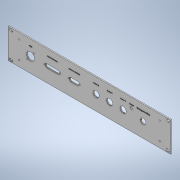
# Autodesk Inventor part: Case_Front
Saved by Autodesk Inventor 2022.2 (Build 262287010, 287A)
## iProperties
Created: 2024-11-06
Part Number: Case_Front
Material: Generisch
Document SubType Name: Modeling
Designer: ppovolni
Density: 1 g/cm^3
Appearance: Vorgabe
Author: ppovolni
Autodesk Inventor part; units mm, degrees
(part 1 of 3)
ref_plane "YZ Plane" through (0, 0, 0) normal (1, 0, 0) x (0, 1, 0)
ref_plane "XZ Plane" through (0, 0, 0) normal (0, 1, 0) x (-1, 0, 0)
ref_plane "XY Plane" through (0, 0, 0) normal (0, 0, 1) x (1, 0, 0)
sketch "Skizze3" plane through (0, 0, 0) normal (0, 0, 1) x (1, 0, 0)
  line L0 (241.3, -44.05) -> (-241.3, -44.05)
  line L1 (-241.3, -44.05) -> (-241.3, 44.05)
  line L2 (-241.3, 44.05) -> (241.3, 44.05)
  line L3 (241.3, 44.05) -> (241.3, -44.05)
  line L4 (241.3, -44.05) -> (-241.3, 44.05) construction
  line L5 (-241.3, -44.05) -> (241.3, 44.05) construction
  line L6 (-233.95, 38.1) -> (-231.05, 38.1) construction
  line L7 (-233.95, 34.35) -> (-231.05, 34.35)
  line L8 (-231.05, 41.85) -> (-233.95, 41.85)
  arc A0 (-233.95, 41.85) -> (-233.95, 34.35) centre (-233.95, 38.1) ccw
  arc A1 (-231.05, 34.35) -> (-231.05, 41.85) centre (-231.05, 38.1) ccw
  line L9 (0, 0) -> (-232.5, 0) construction
  line L10 (-232.5, 0) -> (-232.5, 38.1) construction
  line L11 (-232.5, 38.1) -> (0, 38.1) construction
  line L12 (0, 38.1) -> (0, 0) construction
  line L13 (0, 0) -> (-208.683, 0) construction
  line L14 (-208.683, 0) -> (-208.683, 26.542) construction
  line L15 (-208.683, 26.542) -> (0, 26.542) construction
  line L16 (0, 26.542) -> (0, 0) construction
  circle A2 centre (-208.683, 26.542) radius 1.7
  line L17 (0, 101) -> (0, -128) construction
  line L18 (-346, 0) -> (276, 0) construction
  line L19 (233.95, 34.35) -> (231.05, 34.35)
  line L20 (231.05, 41.85) -> (233.95, 41.85)
  arc A3 (233.95, 34.35) -> (233.95, 41.85) centre (233.95, 38.1) ccw
  arc A4 (231.05, 41.85) -> (231.05, 34.35) centre (231.05, 38.1) ccw
  circle A5 centre (208.683, 26.542) radius 1.7
  line L21 (-233.95, -38.1) -> (-231.05, -38.1) construction
  line L22 (-233.95, -34.35) -> (-231.05, -34.35)
  line L23 (-231.05, -41.85) -> (-233.95, -41.85)
  arc A6 (-233.95, -34.35) -> (-233.95, -41.85) centre (-233.95, -38.1) ccw
  arc A7 (-231.05, -41.85) -> (-231.05, -34.35) centre (-231.05, -38.1) ccw
  circle A8 centre (-208.683, -26.542) radius 1.7
  arc A9 (233.95, -41.85) -> (233.95, -34.35) centre (233.95, -38.1) ccw
  arc A10 (231.05, -34.35) -> (231.05, -41.85) centre (231.05, -38.1) ccw
  line L24 (231.05, -41.85) -> (233.95, -41.85)
  line L25 (233.95, -34.35) -> (231.05, -34.35)
  circle A11 centre (208.683, -26.542) radius 1.7
  point P0 (0, 0)
  point P1 (0, 0)
  point P2 (-227.3, 38.1)
  point P3 (-237.7, 38.1)
  point P4 (-227.3, -38.1)
  point P5 (-237.7, -38.1)
  point P6 (-232.5, -38.1)
  dimension "d0" = 482.6
  dimension "d1" = 88.1
  dimension "d6" = 7.5
  dimension "d7" = 10.4
  dimension "d8" = 38.1
  dimension "d9" = 232.5
  dimension "d10" = 3.4
  dimension "d11" = 208.683
  dimension "d12" = 26.542
  constraints: 56 end point, 25 symmetric about line, 18 point on circle, 12 centre point, 7 parallel, 5 horizontal, 5 midpoint, 4 tangent, 3 perpendicular, 2 coincident, 2 point on line, 1 vertical, 9 other
  measures "d0" distance of L1.end L2.end
  measures "d1" distance of L0.end L1.end
  measures "d6" distance between parallel lines of L7 L8
  measures "d7" distance of point (-227.3, 38.1) point (-237.7, 38.1)
  measures "d8" distance of L9.end L10.end
  measures "d9" distance of L10.end L11.end
  measures "d10" diameter of A2
  measures "d11" distance of L14.end L15.end
  measures "d12" distance of L13.end L14.end
extrude "Extrusion1" add sketch "Skizze3" along normal blind 3
sketch "Skizze4" plane through (0, 0, 3) normal (0, 0, 1) x (1, 0, 0)
  line L0 (241.3, 44.05) -> (-241.3, 44.05) construction
  line L1 (-241.3, 44.05) -> (-241.3, -44.05) construction
  line L2 (-241.3, -44.05) -> (241.3, -44.05) construction
  line L3 (241.3, -44.05) -> (241.3, 44.05) construction
  circle A0 centre (-208.683, 26.542) radius 1.7 construction
  circle A1 centre (208.683, 26.542) radius 1.7 construction
  circle A2 centre (-208.683, -26.542) radius 1.7 construction
  circle A3 centre (208.683, -26.542) radius 1.7 construction
  line L4 (231.05, -34.35) -> (233.95, -34.35) construction
  arc A4 (233.95, -41.85) -> (233.95, -34.35) centre (233.95, -38.1) ccw construction
  line L5 (233.95, -41.85) -> (231.05, -41.85) construction
  arc A5 (231.05, -34.35) -> (231.05, -41.85) centre (231.05, -38.1) ccw construction
  line L6 (-233.95, -34.35) -> (-231.05, -34.35) construction
  arc A6 (-231.05, -41.85) -> (-231.05, -34.35) centre (-231.05, -38.1) ccw construction
  line L7 (-231.05, -41.85) -> (-233.95, -41.85) construction
  arc A7 (-233.95, -34.35) -> (-233.95, -41.85) centre (-233.95, -38.1) ccw construction
  line L8 (231.05, 41.85) -> (233.95, 41.85) construction
  arc A8 (233.95, 34.35) -> (233.95, 41.85) centre (233.95, 38.1) ccw construction
  line L9 (233.95, 34.35) -> (231.05, 34.35) construction
  arc A9 (231.05, 41.85) -> (231.05, 34.35) centre (231.05, 38.1) ccw construction
  arc A10 (-233.95, 41.85) -> (-233.95, 34.35) centre (-233.95, 38.1) ccw construction
  line L10 (-233.95, 41.85) -> (-231.05, 41.85) construction
  arc A11 (-231.05, 34.35) -> (-231.05, 41.85) centre (-231.05, 38.1) ccw construction
  line L11 (-231.05, 34.35) -> (-233.95, 34.35) construction
  circle A12 centre (-175, 0) radius 11.8
  line L12 (-184.5, -12) -> (-165.5, -12) construction
  line L13 (-165.5, -12) -> (-165.5, 12) construction
  line L14 (-165.5, 12) -> (-184.5, 12) construction
  line L15 (-184.5, 12) -> (-184.5, -12) construction
  line L16 (-184.5, -12) -> (-165.5, 12) construction
  line L17 (-165.5, -12) -> (-184.5, 12) construction
  circle A13 centre (-165.5, 12) radius 1.55
  circle A14 centre (-184.5, -12) radius 1.55
  line L18 (-128.2985, 5) -> (-91.7015, 5)
  line L19 (-89.2395, 2.0659) -> (-90.1211, -2.9341)
  line L20 (-92.5832, -5) -> (-127.4168, -5)
  line L21 (-129.8789, -2.9341) -> (-130.7605, 2.0659)
  line L22 (-131.2779, 5) -> (-88.7221, 5) construction
  line L23 (-88.7221, 5) -> (-88.7221, -5) construction
  line L24 (-88.7221, -5) -> (-131.2779, -5) construction
  line L25 (-131.2779, -5) -> (-131.2779, 5) construction
  line L26 (-110, -5) -> (-110, 5) construction
  line L27 (-131.2779, 0) -> (-88.7221, 0) construction
  circle A15 centre (-133.52, 0) radius 1.55
  circle A16 centre (-86.48, 0) radius 1.55
  arc A17 (-128.2985, 5) -> (-130.7605, 2.0659) centre (-128.2985, 2.5) ccw
  arc A18 (-129.8789, -2.9341) -> (-127.4168, -5) centre (-127.4168, -2.5) ccw
  arc A19 (-89.2395, 2.0659) -> (-91.7015, 5) centre (-91.7015, 2.5) ccw
  arc A20 (-92.5832, -5) -> (-90.1211, -2.9341) centre (-92.5832, -2.5) ccw
  line L28 (-56.638, 5.6) -> (-33.362, 5.6)
  line L29 (-30.9, 2.6659) -> (-31.9932, -3.5341)
  line L30 (-34.4552, -5.6) -> (-55.5448, -5.6)
  line L31 (-58.0068, -3.5341) -> (-59.1, 2.6659)
  line L32 (-59.6174, 5.6) -> (-30.3826, 5.6) construction
  line L33 (-30.3826, 5.6) -> (-30.3826, -5.6) construction
  line L34 (-30.3826, -5.6) -> (-59.6174, -5.6) construction
  line L35 (-59.6174, -5.6) -> (-59.6174, 5.6) construction
  line L36 (-45, -5.6) -> (-45, 5.6) construction
  line L37 (-59.6174, 0) -> (-30.3826, 0) construction
  circle A21 centre (-61.66, 0) radius 1.55
  circle A22 centre (-28.34, 0) radius 1.55
  arc A23 (-56.638, 5.6) -> (-59.1, 2.6659) centre (-56.638, 3.1) ccw
  arc A24 (-58.0068, -3.5341) -> (-55.5448, -5.6) centre (-55.5448, -3.1) ccw
  arc A25 (-30.9, 2.6659) -> (-33.362, 5.6) centre (-33.362, 3.1) ccw
  arc A26 (-34.4552, -5.6) -> (-31.9932, -3.5341) centre (-34.4552, -3.1) ccw
  arc A27 (21.536, -8.868) -> (18.464, -8.868) centre (20, 0) ccw
  line L38 (20, 9.0139) -> (20, -9.0139) construction
  line L39 (11, 0) -> (29, 0) construction
  line L40 (20, -8.2) -> (20, -10.3) construction
  arc A28 (21.536, -8.868) -> (18.464, -8.868) centre (20, -10.3) ccw
  arc A29 (61.536, -8.868) -> (58.464, -8.868) centre (60, 0) ccw
  line L41 (60, 31.8347) -> (60, -31.8347) construction
  line L42 (51, 0) -> (69, 0) construction
  line L43 (60, -8.2) -> (60, -10.3) construction
  arc A30 (61.536, -8.868) -> (58.464, -8.868) centre (60, -10.3) ccw
  arc A31 (101.536, -8.868) -> (98.464, -8.868) centre (100, 0) ccw
  line L44 (100, 22.1437) -> (100, -22.1437) construction
  line L45 (91, 0) -> (109, 0) construction
  line L46 (100, -8.2) -> (100, -10.3) construction
  arc A32 (101.536, -8.868) -> (98.464, -8.868) centre (100, -10.3) ccw
  circle A33 centre (125, 17) radius 4
  line L47 (-241.3, 19.05) -> (241.3, 19.05) construction
  line L48 (-180, 19.05) -> (-170, 19.05) construction
  line L49 (-170, 19.05) -> (-170, 24.05) construction
  line L50 (-170, 24.05) -> (-180, 24.05) construction
  line L51 (-180, 24.05) -> (-180, 19.05) construction
  line L52 (-115, 19.05) -> (-105, 19.05) construction
  line L53 (-105, 19.05) -> (-105, 24.05) construction
  line L54 (-105, 24.05) -> (-115, 24.05) construction
  line L55 (-115, 24.05) -> (-115, 19.05) construction
  line L56 (-50, 19.05) -> (-40, 19.05) construction
  line L57 (-40, 19.05) -> (-40, 24.05) construction
  line L58 (-40, 24.05) -> (-50, 24.05) construction
  line L59 (-50, 24.05) -> (-50, 19.05) construction
  line L60 (15, 19.05) -> (25, 19.05) construction
  line L61 (25, 19.05) -> (25, 24.05) construction
  line L62 (25, 24.05) -> (15, 24.05) construction
  line L63 (15, 24.05) -> (15, 19.05) construction
  line L64 (55, 19.05) -> (65, 19.05) construction
  line L65 (65, 19.05) -> (65, 24.05) construction
  line L66 (65, 24.05) -> (55, 24.05) construction
  line L67 (55, 24.05) -> (55, 19.05) construction
  line L68 (95, 19.05) -> (105, 19.05) construction
  line L69 (105, 19.05) -> (105, 24.05) construction
  line L70 (105, 24.05) -> (95, 24.05) construction
  line L71 (95, 24.05) -> (95, 19.05) construction
  line L72 (120, 19.05) -> (130, 19.05) construction
  line L73 (130, 19.05) -> (130, 24.05) construction
  line L74 (130, 24.05) -> (120, 24.05) construction
  line L75 (120, 24.05) -> (120, 19.05) construction
  arc A34 (151.5453, -0.85) -> (151.5453, 0.85) centre (159.5, 0) ccw
  line L76 (152.5, 0) -> (167.5, 0) construction
  line L77 (167.4657, 0.7397) -> (167.4657, -0.7397) construction
  line L78 (151.5453, 0.85) -> (152.5, 0.85)
  line L79 (152.5, 0.85) -> (152.5, -0.85)
  line L80 (152.5, -0.85) -> (151.5453, -0.85)
  line L81 (155, 19.05) -> (165, 19.05) construction
  line L82 (165, 19.05) -> (165, 24.05) construction
  line L83 (165, 24.05) -> (155, 24.05) construction
  line L84 (155, 24.05) -> (155, 19.05) construction
  spline S0 degree 2 poles (-177.7216, 23.9868) (-178.327, 23.9868) (-178.9785, 24.5703) (-178.9785, 25.1343) knots 0 0 0 1 2 2 2
  line L85 (-178.9785, 25.1343) -> (-178.9785, 27.05)
  line L86 (-178.9785, 27.05) -> (-178.2249, 27.05)
  line L87 (-178.2249, 27.05) -> (-178.2249, 25.178)
  spline S1 degree 2 poles (-178.2249, 25.178) (-178.2249, 24.8644) (-177.9891, 24.5581) (-177.7216, 24.5581) knots 0 0 0 1 2 2 2
  spline S2 degree 2 poles (-177.7216, 24.5581) (-177.4615, 24.5581) (-177.2184, 24.8523) (-177.2184, 25.178) knots 0 0 0 1 2 2 2
  line L88 (-177.2184, 25.178) -> (-177.2184, 27.05)
  line L89 (-177.2184, 27.05) -> (-176.4647, 27.05)
  line L90 (-176.4647, 27.05) -> (-176.4647, 25.1367)
  spline S3 degree 2 poles (-176.4647, 25.1367) (-176.4647, 24.5824) (-177.0993, 23.9868) (-177.7216, 23.9868) knots 0 0 0 1 2 2 2
  spline S4 degree 2 poles (-174.9599, 23.9965) (-175.3051, 23.9965) (-175.8254, 24.1302) (-176.049, 24.2275) knots 0 0 0 1 2 2 2
  line L91 (-176.049, 24.2275) -> (-176.049, 24.9422)
  line L92 (-176.049, 24.9422) -> (-175.981, 24.9422)
  spline S5 degree 2 poles (-175.981, 24.9422) (-175.7549, 24.7502) (-175.2127, 24.5435) (-174.9575, 24.5435) knots 0 0 0 1 2 2 2
  spline S6 degree 2 poles (-174.9575, 24.5435) (-174.8918, 24.5435) (-174.6803, 24.5727) (-174.6171, 24.6019) knots 0 0 0 1 2 2 2
  spline S7 degree 2 poles (-174.6171, 24.6019) (-174.5393, 24.6359) (-174.4299, 24.7599) (-174.4299, 24.8596) knots 0 0 0 1 2 2 2
  spline S8 degree 2 poles (-174.4299, 24.8596) (-174.4299, 24.9738) (-174.6074, 25.1148) (-174.7289, 25.1464) knots 0 0 0 1 2 2 2
  spline S9 degree 2 poles (-174.7289, 25.1464) (-174.8821, 25.1878) (-175.2297, 25.2583) (-175.3829, 25.3118) knots 0 0 0 1 2 2 2
  spline S10 degree 2 poles (-175.3829, 25.3118) (-175.7306, 25.4333) (-176.032, 25.849) (-176.032, 26.1602) knots 0 0 0 1 2 2 2
  spline S11 degree 2 poles (-176.032, 26.1602) (-176.032, 26.5808) (-175.3197, 27.1035) (-174.7848, 27.1035) knots 0 0 0 1 2 2 2
  spline S12 degree 2 poles (-174.7848, 27.1035) (-174.5174, 27.1035) (-173.9874, 26.9941) (-173.7784, 26.9017) knots 0 0 0 1 2 2 2
  line L93 (-173.7784, 26.9017) -> (-173.7784, 26.2161)
  line L94 (-173.7784, 26.2161) -> (-173.844, 26.2161)
  spline S13 degree 2 poles (-173.844, 26.2161) (-174.0118, 26.3596) (-174.4931, 26.5565) (-174.7459, 26.5565) knots 0 0 0 1 2 2 2
  spline S14 degree 2 poles (-174.7459, 26.5565) (-174.8456, 26.5565) (-175.0012, 26.5273) (-175.0887, 26.4884) knots 0 0 0 1 2 2 2
  spline S15 degree 2 poles (-175.0887, 26.4884) (-175.1592, 26.4568) (-175.2613, 26.3304) (-175.2613, 26.2526) knots 0 0 0 1 2 2 2
  spline S16 degree 2 poles (-175.2613, 26.2526) (-175.2613, 26.1359) (-175.0985, 26.0022) (-174.8651, 25.9487) knots 0 0 0 1 2 2 2
  spline S17 degree 2 poles (-174.8651, 25.9487) (-174.7143, 25.9147) (-174.4348, 25.849) (-174.2743, 25.7931) knots 0 0 0 1 2 2 2
  spline S18 degree 2 poles (-174.2743, 25.7931) (-173.9631, 25.6788) (-173.6592, 25.2996) (-173.6592, 24.9884) knots 0 0 0 1 2 2 2
  spline S19 degree 2 poles (-173.6592, 24.9884) (-173.6592, 24.5411) (-174.3618, 23.9965) (-174.9599, 23.9965) knots 0 0 0 1 2 2 2
  spline S20 degree 2 poles (-170.8756, 24.969) (-170.8756, 24.7453) (-171.0458, 24.4074) (-171.1868, 24.2955) knots 0 0 0 1 2 2 2
  spline S21 degree 2 poles (-171.1868, 24.2955) (-171.357, 24.1618) (-171.7605, 24.05) (-172.0741, 24.05) knots 0 0 0 1 2 2 2
  line L95 (-172.0741, 24.05) -> (-173.2727, 24.05)
  line L96 (-173.2727, 24.05) -> (-173.2727, 27.05)
  line L97 (-173.2727, 27.05) -> (-172.2152, 27.05)
  spline S22 degree 2 poles (-172.2152, 27.05) (-171.8845, 27.05) (-171.5442, 26.9989) (-171.3959, 26.9187) knots 0 0 0 1 2 2 2
  spline S23 degree 2 poles (-171.3959, 26.9187) (-171.233, 26.8336) (-171.075, 26.5419) (-171.075, 26.3523) knots 0 0 0 1 2 2 2
  spline S24 degree 2 poles (-171.075, 26.3523) (-171.075, 26.1335) (-171.2938, 25.7907) (-171.4882, 25.7105) knots 0 0 0 1 2 2 2
  line L98 (-171.4882, 25.7105) -> (-171.4882, 25.6959)
  spline S25 degree 2 poles (-171.4882, 25.6959) (-171.2087, 25.6375) (-170.8756, 25.2753) (-170.8756, 24.969) knots 0 0 0 1 2 2 2
  spline S26 degree 2 poles (-171.6536, 24.9811) (-171.6536, 25.1221) (-171.7654, 25.2801) (-171.8772, 25.3215) knots 0 0 0 1 2 2 2
  spline S27 degree 2 poles (-171.8772, 25.3215) (-171.9453, 25.3482) (-172.186, 25.3531) (-172.3853, 25.3531) knots 0 0 0 1 2 2 2
  line L99 (-172.3853, 25.3531) -> (-172.5239, 25.3531)
  line L100 (-172.5239, 25.3531) -> (-172.5239, 24.597)
  line L101 (-172.5239, 24.597) -> (-172.4826, 24.597)
  spline S28 degree 2 poles (-172.4826, 24.597) (-172.1908, 24.597) (-171.9672, 24.6043) (-171.8505, 24.6553) knots 0 0 0 1 2 2 2
  spline S29 degree 2 poles (-171.8505, 24.6553) (-171.7484, 24.7015) (-171.6536, 24.8717) (-171.6536, 24.9811) knots 0 0 0 1 2 2 2
  spline S30 degree 2 poles (-171.8408, 26.204) (-171.8408, 26.2769) (-171.9161, 26.4301) (-171.9939, 26.4641) knots 0 0 0 1 2 2 2
  spline S31 degree 2 poles (-171.9939, 26.4641) (-172.0669, 26.4981) (-172.2711, 26.503) (-172.4729, 26.503) knots 0 0 0 1 2 2 2
  line L102 (-172.4729, 26.503) -> (-172.5239, 26.503)
  line L103 (-172.5239, 26.503) -> (-172.5239, 25.866)
  line L104 (-172.5239, 25.866) -> (-172.4291, 25.866)
  spline S32 degree 2 poles (-172.4291, 25.866) (-172.237, 25.866) (-172.0814, 25.8733) (-171.9988, 25.9122) knots 0 0 0 1 2 2 2
  spline S33 degree 2 poles (-171.9988, 25.9122) (-171.9088, 25.956) (-171.8408, 26.1043) (-171.8408, 26.204) knots 0 0 0 1 2 2 2
  line L105 (-122.857, 24.05) -> (-124.8578, 24.05)
  line L106 (-124.8578, 24.05) -> (-124.8578, 27.05)
  line L107 (-124.8578, 27.05) -> (-124.1041, 27.05)
  line L108 (-124.1041, 27.05) -> (-124.1041, 24.6213)
  line L109 (-124.1041, 24.6213) -> (-122.857, 24.6213)
  line L110 (-122.857, 24.6213) -> (-122.857, 24.05)
  line L111 (-121.8335, 24.05) -> (-122.5385, 24.05)
  line L112 (-122.5385, 24.05) -> (-122.5385, 26.3134)
  line L113 (-122.5385, 26.3134) -> (-121.8335, 26.3134)
  line L114 (-121.8335, 26.3134) -> (-121.8335, 24.05)
  line L115 (-121.8116, 26.6367) -> (-122.5579, 26.6367)
  line L116 (-122.5579, 26.6367) -> (-122.5579, 27.1861)
  line L117 (-122.5579, 27.1861) -> (-121.8116, 27.1861)
  line L118 (-121.8116, 27.1861) -> (-121.8116, 26.6367)
  line L119 (-118.5928, 24.05) -> (-118.5928, 25.1805)
  spline S34 degree 2 poles (-118.5928, 25.1805) (-118.5928, 25.3482) (-118.6049, 25.5767) (-118.6341, 25.6497) knots 0 0 0 1 2 2 2
  spline S35 degree 2 poles (-118.6341, 25.6497) (-118.6657, 25.7226) (-118.7921, 25.7882) (-118.9064, 25.7882) knots 0 0 0 1 2 2 2
  spline S36 degree 2 poles (-118.9064, 25.7882) (-118.9866, 25.7882) (-119.1422, 25.7177) (-119.2346, 25.6521) knots 0 0 0 1 2 2 2
  line L120 (-119.2346, 25.6521) -> (-119.2346, 24.05)
  line L121 (-119.2346, 24.05) -> (-119.9445, 24.05)
  line L122 (-119.9445, 24.05) -> (-119.9445, 25.1805)
  spline S37 degree 2 poles (-119.9445, 25.1805) (-119.9445, 25.3458) (-119.9591, 25.5767) (-119.9883, 25.6497) knots 0 0 0 1 2 2 2
  spline S38 degree 2 poles (-119.9883, 25.6497) (-120.0199, 25.7226) (-120.1463, 25.7882) (-120.2605, 25.7882) knots 0 0 0 1 2 2 2
  spline S39 degree 2 poles (-120.2605, 25.7882) (-120.3456, 25.7882) (-120.5134, 25.708) (-120.5912, 25.6521) knots 0 0 0 1 2 2 2
  line L123 (-120.5912, 25.6521) -> (-120.5912, 24.05)
  line L124 (-120.5912, 24.05) -> (-121.2962, 24.05)
  line L125 (-121.2962, 24.05) -> (-121.2962, 26.3134)
  line L126 (-121.2962, 26.3134) -> (-120.5912, 26.3134)
  line L127 (-120.5912, 26.3134) -> (-120.5912, 26.063)
  spline S40 degree 2 poles (-120.5912, 26.063) (-120.4186, 26.2088) (-120.1098, 26.3741) (-119.9177, 26.3741) knots 0 0 0 1 2 2 2
  spline S41 degree 2 poles (-119.9177, 26.3741) (-119.7111, 26.3741) (-119.3951, 26.1772) (-119.3124, 25.9803) knots 0 0 0 1 2 2 2
  spline S42 degree 2 poles (-119.3124, 25.9803) (-119.1106, 26.1699) (-118.7508, 26.3741) (-118.566, 26.3741) knots 0 0 0 1 2 2 2
  spline S43 degree 2 poles (-118.566, 26.3741) (-118.408, 26.3741) (-118.1576, 26.2745) (-118.0725, 26.1724) knots 0 0 0 1 2 2 2
  spline S44 degree 2 poles (-118.0725, 26.1724) (-117.9777, 26.063) (-117.8829, 25.7639) (-117.8829, 25.5233) knots 0 0 0 1 2 2 2
  line L128 (-117.8829, 25.5233) -> (-117.8829, 24.05)
  line L129 (-117.8829, 24.05) -> (-118.5928, 24.05)
  line L130 (-116.6552, 24.05) -> (-117.3602, 24.05)
  line L131 (-117.3602, 24.05) -> (-117.3602, 26.3134)
  line L132 (-117.3602, 26.3134) -> (-116.6552, 26.3134)
  line L133 (-116.6552, 26.3134) -> (-116.6552, 24.05)
  line L134 (-116.6333, 26.6367) -> (-117.3797, 26.6367)
  line L135 (-117.3797, 26.6367) -> (-117.3797, 27.1861)
  line L136 (-117.3797, 27.1861) -> (-116.6333, 27.1861)
  line L137 (-116.6333, 27.1861) -> (-116.6333, 26.6367)
  spline S45 degree 2 poles (-115.25, 24.0062) (-115.6803, 24.0062) (-116.0741, 24.3612) (-116.0741, 24.7647) knots 0 0 0 1 2 2 2
  line L138 (-116.0741, 24.7647) -> (-116.0741, 25.8223)
  line L139 (-116.0741, 25.8223) -> (-116.344, 25.8223)
  line L140 (-116.344, 25.8223) -> (-116.344, 26.3134)
  line L141 (-116.344, 26.3134) -> (-116.0741, 26.3134)
  line L142 (-116.0741, 26.3134) -> (-116.0741, 26.96)
  line L143 (-116.0741, 26.96) -> (-115.3691, 26.96)
  line L144 (-115.3691, 26.96) -> (-115.3691, 26.3134)
  line L145 (-115.3691, 26.3134) -> (-114.6884, 26.3134)
  line L146 (-114.6884, 26.3134) -> (-114.6884, 25.8223)
  line L147 (-114.6884, 25.8223) -> (-115.3691, 25.8223)
  line L148 (-115.3691, 25.8223) -> (-115.3691, 25.0176)
  spline S46 degree 2 poles (-115.3691, 25.0176) (-115.3691, 24.8985) (-115.3643, 24.721) (-115.3351, 24.6505) knots 0 0 0 1 2 2 2
  spline S47 degree 2 poles (-115.3351, 24.6505) (-115.3059, 24.58) (-115.1625, 24.4973) (-115.0263, 24.4973) knots 0 0 0 1 2 2 2
  spline S48 degree 2 poles (-115.0263, 24.4973) (-114.968, 24.4973) (-114.7857, 24.5459) (-114.7492, 24.5654) knots 0 0 0 1 2 2 2
  line L149 (-114.7492, 24.5654) -> (-114.6884, 24.5654)
  line L150 (-114.6884, 24.5654) -> (-114.6884, 24.0694)
  spline S49 degree 2 poles (-114.6884, 24.0694) (-114.8027, 24.0403) (-115.0604, 24.0062) (-115.25, 24.0062) knots 0 0 0 1 2 2 2
  spline S50 degree 2 poles (-112.2257, 23.9965) (-112.5709, 23.9965) (-113.0912, 24.1302) (-113.3148, 24.2275) knots 0 0 0 1 2 2 2
  line L151 (-113.3148, 24.2275) -> (-113.3148, 24.9422)
  line L152 (-113.3148, 24.9422) -> (-113.2468, 24.9422)
  spline S51 degree 2 poles (-113.2468, 24.9422) (-113.0207, 24.7502) (-112.4785, 24.5435) (-112.2233, 24.5435) knots 0 0 0 1 2 2 2
  spline S52 degree 2 poles (-112.2233, 24.5435) (-112.1576, 24.5435) (-111.9461, 24.5727) (-111.8829, 24.6019) knots 0 0 0 1 2 2 2
  spline S53 degree 2 poles (-111.8829, 24.6019) (-111.8051, 24.6359) (-111.6957, 24.7599) (-111.6957, 24.8596) knots 0 0 0 1 2 2 2
  spline S54 degree 2 poles (-111.6957, 24.8596) (-111.6957, 24.9738) (-111.8732, 25.1148) (-111.9947, 25.1464) knots 0 0 0 1 2 2 2
  spline S55 degree 2 poles (-111.9947, 25.1464) (-112.1479, 25.1878) (-112.4955, 25.2583) (-112.6487, 25.3118) knots 0 0 0 1 2 2 2
  spline S56 degree 2 poles (-112.6487, 25.3118) (-112.9964, 25.4333) (-113.2978, 25.849) (-113.2978, 26.1602) knots 0 0 0 1 2 2 2
  spline S57 degree 2 poles (-113.2978, 26.1602) (-113.2978, 26.5808) (-112.5855, 27.1035) (-112.0506, 27.1035) knots 0 0 0 1 2 2 2
  spline S58 degree 2 poles (-112.0506, 27.1035) (-111.7832, 27.1035) (-111.2532, 26.9941) (-111.0442, 26.9017) knots 0 0 0 1 2 2 2
  line L153 (-111.0442, 26.9017) -> (-111.0442, 26.2161)
  line L154 (-111.0442, 26.2161) -> (-111.1098, 26.2161)
  spline S59 degree 2 poles (-111.1098, 26.2161) (-111.2776, 26.3596) (-111.7589, 26.5565) (-112.0118, 26.5565) knots 0 0 0 1 2 2 2
  spline S60 degree 2 poles (-112.0118, 26.5565) (-112.1114, 26.5565) (-112.267, 26.5273) (-112.3545, 26.4884) knots 0 0 0 1 2 2 2
  spline S61 degree 2 poles (-112.3545, 26.4884) (-112.425, 26.4568) (-112.5271, 26.3304) (-112.5271, 26.2526) knots 0 0 0 1 2 2 2
  spline S62 degree 2 poles (-112.5271, 26.2526) (-112.5271, 26.1359) (-112.3643, 26.0022) (-112.1309, 25.9487) knots 0 0 0 1 2 2 2
  spline S63 degree 2 poles (-112.1309, 25.9487) (-111.9801, 25.9147) (-111.7006, 25.849) (-111.5401, 25.7931) knots 0 0 0 1 2 2 2
  spline S64 degree 2 poles (-111.5401, 25.7931) (-111.2289, 25.6788) (-110.925, 25.2996) (-110.925, 24.9884) knots 0 0 0 1 2 2 2
  spline S65 degree 2 poles (-110.925, 24.9884) (-110.925, 24.5411) (-111.6276, 23.9965) (-112.2257, 23.9965) knots 0 0 0 1 2 2 2
  line L155 (-107.2079, 26.3134) -> (-107.8691, 24.05)
  line L156 (-107.8691, 24.05) -> (-108.6179, 24.05)
  line L157 (-108.6179, 24.05) -> (-109.0166, 25.5135)
  line L158 (-109.0166, 25.5135) -> (-109.4153, 24.05)
  line L159 (-109.4153, 24.05) -> (-110.1641, 24.05)
  line L160 (-110.1641, 24.05) -> (-110.8205, 26.3134)
  line L161 (-110.8205, 26.3134) -> (-110.079, 26.3134)
  line L162 (-110.079, 26.3134) -> (-109.7314, 24.8158)
  line L163 (-109.7314, 24.8158) -> (-109.3035, 26.3134)
  line L164 (-109.3035, 26.3134) -> (-108.6787, 26.3134)
  line L165 (-108.6787, 26.3134) -> (-108.2751, 24.8158)
  line L166 (-108.2751, 24.8158) -> (-107.9323, 26.3134)
  line L167 (-107.9323, 26.3134) -> (-107.2079, 26.3134)
  line L168 (-106.2038, 24.05) -> (-106.9088, 24.05)
  line L169 (-106.9088, 24.05) -> (-106.9088, 26.3134)
  line L170 (-106.9088, 26.3134) -> (-106.2038, 26.3134)
  line L171 (-106.2038, 26.3134) -> (-106.2038, 24.05)
  line L172 (-106.1819, 26.6367) -> (-106.9283, 26.6367)
  line L173 (-106.9283, 26.6367) -> (-106.9283, 27.1861)
  line L174 (-106.9283, 27.1861) -> (-106.1819, 27.1861)
  line L175 (-106.1819, 27.1861) -> (-106.1819, 26.6367)
  spline S66 degree 2 poles (-104.7986, 24.0062) (-105.2289, 24.0062) (-105.6228, 24.3612) (-105.6228, 24.7647) knots 0 0 0 1 2 2 2
  line L176 (-105.6228, 24.7647) -> (-105.6228, 25.8223)
  line L177 (-105.6228, 25.8223) -> (-105.8926, 25.8223)
  line L178 (-105.8926, 25.8223) -> (-105.8926, 26.3134)
  line L179 (-105.8926, 26.3134) -> (-105.6228, 26.3134)
  line L180 (-105.6228, 26.3134) -> (-105.6228, 26.96)
  line L181 (-105.6228, 26.96) -> (-104.9177, 26.96)
  line L182 (-104.9177, 26.96) -> (-104.9177, 26.3134)
  line L183 (-104.9177, 26.3134) -> (-104.237, 26.3134)
  line L184 (-104.237, 26.3134) -> (-104.237, 25.8223)
  line L185 (-104.237, 25.8223) -> (-104.9177, 25.8223)
  line L186 (-104.9177, 25.8223) -> (-104.9177, 25.0176)
  spline S67 degree 2 poles (-104.9177, 25.0176) (-104.9177, 24.8985) (-104.9129, 24.721) (-104.8837, 24.6505) knots 0 0 0 1 2 2 2
  spline S68 degree 2 poles (-104.8837, 24.6505) (-104.8545, 24.58) (-104.7111, 24.4973) (-104.575, 24.4973) knots 0 0 0 1 2 2 2
  spline S69 degree 2 poles (-104.575, 24.4973) (-104.5166, 24.4973) (-104.3343, 24.5459) (-104.2978, 24.5654) knots 0 0 0 1 2 2 2
  line L187 (-104.2978, 24.5654) -> (-104.237, 24.5654)
  line L188 (-104.237, 24.5654) -> (-104.237, 24.0694)
  spline S70 degree 2 poles (-104.237, 24.0694) (-104.3513, 24.0403) (-104.609, 24.0062) (-104.7986, 24.0062) knots 0 0 0 1 2 2 2
  spline S71 degree 2 poles (-102.8416, 23.9892) (-103.1211, 23.9892) (-103.5855, 24.1302) (-103.7581, 24.2761) knots 0 0 0 1 2 2 2
  spline S72 degree 2 poles (-103.7581, 24.2761) (-103.9259, 24.4244) (-104.1155, 24.8693) (-104.1155, 25.1707) knots 0 0 0 1 2 2 2
  spline S73 degree 2 poles (-104.1155, 25.1707) (-104.1155, 25.4965) (-103.9113, 25.9511) (-103.7338, 26.097) knots 0 0 0 1 2 2 2
  spline S74 degree 2 poles (-103.7338, 26.097) (-103.566, 26.238) (-103.109, 26.3741) (-102.861, 26.3741) knots 0 0 0 1 2 2 2
  spline S75 degree 2 poles (-102.861, 26.3741) (-102.6738, 26.3741) (-102.2994, 26.2866) (-102.1098, 26.1918) knots 0 0 0 1 2 2 2
  line L189 (-102.1098, 26.1918) -> (-102.1098, 25.5889)
  line L190 (-102.1098, 25.5889) -> (-102.1998, 25.5889)
  spline S76 degree 2 poles (-102.1998, 25.5889) (-102.2435, 25.6302) (-102.3651, 25.7275) (-102.438, 25.7664) knots 0 0 0 1 2 2 2
  spline S77 degree 2 poles (-102.438, 25.7664) (-102.5158, 25.8101) (-102.7079, 25.8685) (-102.827, 25.8685) knots 0 0 0 1 2 2 2
  spline S78 degree 2 poles (-102.827, 25.8685) (-103.0968, 25.8685) (-103.3934, 25.4917) (-103.3934, 25.1707) knots 0 0 0 1 2 2 2
  spline S79 degree 2 poles (-103.3934, 25.1707) (-103.3934, 24.8304) (-103.0774, 24.4949) (-102.8148, 24.4949) knots 0 0 0 1 2 2 2
  spline S80 degree 2 poles (-102.8148, 24.4949) (-102.6811, 24.4949) (-102.4818, 24.5557) (-102.4088, 24.5994) knots 0 0 0 1 2 2 2
  spline S81 degree 2 poles (-102.4088, 24.5994) (-102.3383, 24.6408) (-102.2362, 24.7331) (-102.1998, 24.7696) knots 0 0 0 1 2 2 2
  line L191 (-102.1998, 24.7696) -> (-102.1098, 24.7696)
  line L192 (-102.1098, 24.7696) -> (-102.1098, 24.1643)
  spline S82 degree 2 poles (-102.1098, 24.1643) (-102.1706, 24.1375) (-102.3286, 24.0694) (-102.4113, 24.0476) knots 0 0 0 1 2 2 2
  spline S83 degree 2 poles (-102.4113, 24.0476) (-102.5134, 24.0184) (-102.6933, 23.9892) (-102.8416, 23.9892) knots 0 0 0 1 2 2 2
  line L193 (-99.6568, 24.05) -> (-100.3667, 24.05)
  line L194 (-100.3667, 24.05) -> (-100.3667, 25.1707)
  spline S84 degree 2 poles (-100.3667, 25.1707) (-100.3667, 25.3093) (-100.3886, 25.5816) (-100.4177, 25.6448) knots 0 0 0 1 2 2 2
  spline S85 degree 2 poles (-100.4177, 25.6448) (-100.4542, 25.7226) (-100.5904, 25.7882) (-100.707, 25.7882) knots 0 0 0 1 2 2 2
  spline S86 degree 2 poles (-100.707, 25.7882) (-100.7921, 25.7882) (-100.9696, 25.7226) (-101.0693, 25.6521) knots 0 0 0 1 2 2 2
  line L195 (-101.0693, 25.6521) -> (-101.0693, 24.05)
  line L196 (-101.0693, 24.05) -> (-101.7743, 24.05)
  line L197 (-101.7743, 24.05) -> (-101.7743, 27.1837)
  line L198 (-101.7743, 27.1837) -> (-101.0693, 27.1837)
  line L199 (-101.0693, 27.1837) -> (-101.0693, 26.063)
  spline S87 degree 2 poles (-101.0693, 26.063) (-100.8967, 26.2088) (-100.5685, 26.3741) (-100.3691, 26.3741) knots 0 0 0 1 2 2 2
  spline S88 degree 2 poles (-100.3691, 26.3741) (-100.0239, 26.3741) (-99.6568, 25.9365) (-99.6568, 25.5233) knots 0 0 0 1 2 2 2
  line L200 (-99.6568, 25.5233) -> (-99.6568, 24.05)
  spline S89 degree 2 poles (-97.9745, 23.9892) (-98.6163, 23.9892) (-99.2994, 24.6019) (-99.2994, 25.1683) knots 0 0 0 1 2 2 2
  spline S90 degree 2 poles (-99.2994, 25.1683) (-99.2994, 25.7226) (-98.6625, 26.3839) (-98.0887, 26.3839) knots 0 0 0 1 2 2 2
  spline S91 degree 2 poles (-98.0887, 26.3839) (-97.5709, 26.3839) (-97.0458, 25.8223) (-97.0458, 25.302) knots 0 0 0 1 2 2 2
  line L201 (-97.0458, 25.302) -> (-97.0458, 25.0468)
  line L202 (-97.0458, 25.0468) -> (-98.5944, 25.0468)
  spline S92 degree 2 poles (-98.5944, 25.0468) (-98.5847, 24.8887) (-98.4704, 24.6797) (-98.378, 24.6165) knots 0 0 0 1 2 2 2
  spline S93 degree 2 poles (-98.378, 24.6165) (-98.2881, 24.5532) (-98.045, 24.4998) (-97.9015, 24.4998) knots 0 0 0 1 2 2 2
  spline S94 degree 2 poles (-97.9015, 24.4998) (-97.78, 24.4998) (-97.5417, 24.5532) (-97.4421, 24.5994) knots 0 0 0 1 2 2 2
  spline S95 degree 2 poles (-97.4421, 24.5994) (-97.3545, 24.6359) (-97.2087, 24.7259) (-97.1625, 24.7599) knots 0 0 0 1 2 2 2
  line L203 (-97.1625, 24.7599) -> (-97.0871, 24.7599)
  line L204 (-97.0871, 24.7599) -> (-97.0871, 24.1764)
  spline S96 degree 2 poles (-97.0871, 24.1764) (-97.1746, 24.1424) (-97.3156, 24.084) (-97.4421, 24.0549) knots 0 0 0 1 2 2 2
  spline S97 degree 2 poles (-97.4421, 24.0549) (-97.5563, 24.0233) (-97.7994, 23.9892) (-97.9745, 23.9892) knots 0 0 0 1 2 2 2
  spline S98 degree 2 poles (-97.7411, 25.4722) (-97.7459, 25.6959) (-97.9429, 25.9317) (-98.1447, 25.9317) knots 0 0 0 1 2 2 2
  spline S99 degree 2 poles (-98.1447, 25.9317) (-98.3513, 25.9317) (-98.5847, 25.6837) (-98.5968, 25.4722) knots 0 0 0 1 2 2 2
  line L205 (-98.5968, 25.4722) -> (-97.7411, 25.4722)
  spline S100 degree 2 poles (-95.9955, 23.9892) (-96.2435, 23.9892) (-96.6884, 24.0986) (-96.8343, 24.1716) knots 0 0 0 1 2 2 2
  line L206 (-96.8343, 24.1716) -> (-96.8343, 24.7672)
  line L207 (-96.8343, 24.7672) -> (-96.7759, 24.7672)
  spline S101 degree 2 poles (-96.7759, 24.7672) (-96.7249, 24.7283) (-96.596, 24.6359) (-96.4818, 24.5848) knots 0 0 0 1 2 2 2
  spline S102 degree 2 poles (-96.4818, 24.5848) (-96.3821, 24.5387) (-96.1365, 24.473) (-95.9907, 24.473) knots 0 0 0 1 2 2 2
  spline S103 degree 2 poles (-95.9907, 24.473) (-95.8424, 24.473) (-95.6139, 24.5654) (-95.6139, 24.6651) knots 0 0 0 1 2 2 2
  spline S104 degree 2 poles (-95.6139, 24.6651) (-95.6139, 24.7429) (-95.7184, 24.8255) (-95.8691, 24.8596) knots 0 0 0 1 2 2 2
  spline S105 degree 2 poles (-95.8691, 24.8596) (-95.9494, 24.8814) (-96.1949, 24.9276) (-96.2897, 24.9568) knots 0 0 0 1 2 2 2
  spline S106 degree 2 poles (-96.2897, 24.9568) (-96.5571, 25.0395) (-96.8246, 25.3628) (-96.8246, 25.6278) knots 0 0 0 1 2 2 2
  spline S107 degree 2 poles (-96.8246, 25.6278) (-96.8246, 25.7785) (-96.686, 26.0459) (-96.5498, 26.1505) knots 0 0 0 1 2 2 2
  spline S108 degree 2 poles (-96.5498, 26.1505) (-96.4161, 26.2526) (-96.0199, 26.3741) (-95.7694, 26.3741) knots 0 0 0 1 2 2 2
  spline S109 degree 2 poles (-95.7694, 26.3741) (-95.5312, 26.3741) (-95.1325, 26.2793) (-94.9964, 26.2137) knots 0 0 0 1 2 2 2
  line L208 (-94.9964, 26.2137) -> (-94.9964, 25.64)
  line L209 (-94.9964, 25.64) -> (-95.0523, 25.64)
  spline S110 degree 2 poles (-95.0523, 25.64) (-95.0887, 25.6691) (-95.2468, 25.7639) (-95.3197, 25.798) knots 0 0 0 1 2 2 2
  spline S111 degree 2 poles (-95.3197, 25.798) (-95.4096, 25.8369) (-95.6284, 25.8904) (-95.7427, 25.8904) knots 0 0 0 1 2 2 2
  spline S112 degree 2 poles (-95.7427, 25.8904) (-95.8959, 25.8904) (-96.1074, 25.7858) (-96.1074, 25.7007) knots 0 0 0 1 2 2 2
  spline S113 degree 2 poles (-96.1074, 25.7007) (-96.1074, 25.6229) (-96.0028, 25.5354) (-95.8278, 25.4917) knots 0 0 0 1 2 2 2
  spline S114 degree 2 poles (-95.8278, 25.4917) (-95.7378, 25.4698) (-95.502, 25.4284) (-95.3926, 25.392) knots 0 0 0 1 2 2 2
  spline S115 degree 2 poles (-95.3926, 25.392) (-95.1495, 25.3142) (-94.8967, 25.0103) (-94.8967, 24.7575) knots 0 0 0 1 2 2 2
  spline S116 degree 2 poles (-94.8967, 24.7575) (-94.8967, 24.5994) (-95.045, 24.3101) (-95.1835, 24.2129) knots 0 0 0 1 2 2 2
  spline S117 degree 2 poles (-95.1835, 24.2129) (-95.327, 24.1059) (-95.7208, 23.9892) (-95.9955, 23.9892) knots 0 0 0 1 2 2 2
  line L210 (-58.1827, 24.05) -> (-59.0993, 24.05)
  line L211 (-59.0993, 24.05) -> (-59.9331, 25.1513)
  line L212 (-59.9331, 25.1513) -> (-60.2054, 25.1513)
  line L213 (-60.2054, 25.1513) -> (-60.2054, 24.05)
  line L214 (-60.2054, 24.05) -> (-60.9542, 24.05)
  line L215 (-60.9542, 24.05) -> (-60.9542, 27.05)
  line L216 (-60.9542, 27.05) -> (-59.7484, 27.05)
  spline S118 degree 2 poles (-59.7484, 27.05) (-59.498, 27.05) (-59.1284, 26.9868) (-58.9704, 26.8895) knots 0 0 0 1 2 2 2
  spline S119 degree 2 poles (-58.9704, 26.8895) (-58.81, 26.7874) (-58.6203, 26.469) (-58.6203, 26.2259) knots 0 0 0 1 2 2 2
  spline S120 degree 2 poles (-58.6203, 26.2259) (-58.6203, 25.8831) (-58.9315, 25.4528) (-59.1917, 25.3263) knots 0 0 0 1 2 2 2
  line L217 (-59.1917, 25.3263) -> (-58.1827, 24.05)
  spline S121 degree 2 poles (-59.3934, 26.131) (-59.3934, 26.2453) (-59.481, 26.4082) (-59.5806, 26.4519) knots 0 0 0 1 2 2 2
  spline S122 degree 2 poles (-59.5806, 26.4519) (-59.6511, 26.4811) (-59.8237, 26.4981) (-59.9526, 26.4981) knots 0 0 0 1 2 2 2
  line L218 (-59.9526, 26.4981) -> (-60.2054, 26.4981)
  line L219 (-60.2054, 26.4981) -> (-60.2054, 25.691)
  line L220 (-60.2054, 25.691) -> (-59.9891, 25.691)
  spline S123 degree 2 poles (-59.9891, 25.691) (-59.8335, 25.691) (-59.6122, 25.7299) (-59.5369, 25.7907) knots 0 0 0 1 2 2 2
  spline S124 degree 2 poles (-59.5369, 25.7907) (-59.4639, 25.849) (-59.3934, 26.0046) (-59.3934, 26.131) knots 0 0 0 1 2 2 2
  spline S125 degree 2 poles (-56.8408, 23.9892) (-57.4826, 23.9892) (-58.1657, 24.6019) (-58.1657, 25.1683) knots 0 0 0 1 2 2 2
  spline S126 degree 2 poles (-58.1657, 25.1683) (-58.1657, 25.7226) (-57.5288, 26.3839) (-56.955, 26.3839) knots 0 0 0 1 2 2 2
  spline S127 degree 2 poles (-56.955, 26.3839) (-56.4372, 26.3839) (-55.9121, 25.8223) (-55.9121, 25.302) knots 0 0 0 1 2 2 2
  line L221 (-55.9121, 25.302) -> (-55.9121, 25.0468)
  line L222 (-55.9121, 25.0468) -> (-57.4607, 25.0468)
  spline S128 degree 2 poles (-57.4607, 25.0468) (-57.451, 24.8887) (-57.3367, 24.6797) (-57.2443, 24.6165) knots 0 0 0 1 2 2 2
  spline S129 degree 2 poles (-57.2443, 24.6165) (-57.1544, 24.5532) (-56.9113, 24.4998) (-56.7678, 24.4998) knots 0 0 0 1 2 2 2
  spline S130 degree 2 poles (-56.7678, 24.4998) (-56.6463, 24.4998) (-56.408, 24.5532) (-56.3083, 24.5994) knots 0 0 0 1 2 2 2
  spline S131 degree 2 poles (-56.3083, 24.5994) (-56.2208, 24.6359) (-56.075, 24.7259) (-56.0288, 24.7599) knots 0 0 0 1 2 2 2
  line L223 (-56.0288, 24.7599) -> (-55.9534, 24.7599)
  line L224 (-55.9534, 24.7599) -> (-55.9534, 24.1764)
  spline S132 degree 2 poles (-55.9534, 24.1764) (-56.0409, 24.1424) (-56.1819, 24.084) (-56.3083, 24.0549) knots 0 0 0 1 2 2 2
  spline S133 degree 2 poles (-56.3083, 24.0549) (-56.4226, 24.0233) (-56.6657, 23.9892) (-56.8408, 23.9892) knots 0 0 0 1 2 2 2
  spline S134 degree 2 poles (-56.6074, 25.4722) (-56.6122, 25.6959) (-56.8092, 25.9317) (-57.0109, 25.9317) knots 0 0 0 1 2 2 2
  spline S135 degree 2 poles (-57.0109, 25.9317) (-57.2176, 25.9317) (-57.451, 25.6837) (-57.4631, 25.4722) knots 0 0 0 1 2 2 2
  line L225 (-57.4631, 25.4722) -> (-56.6074, 25.4722)
  line L226 (-52.8489, 24.05) -> (-52.8489, 25.1805)
  spline S136 degree 2 poles (-52.8489, 25.1805) (-52.8489, 25.3482) (-52.861, 25.5767) (-52.8902, 25.6497) knots 0 0 0 1 2 2 2
  spline S137 degree 2 poles (-52.8902, 25.6497) (-52.9218, 25.7226) (-53.0482, 25.7882) (-53.1625, 25.7882) knots 0 0 0 1 2 2 2
  spline S138 degree 2 poles (-53.1625, 25.7882) (-53.2427, 25.7882) (-53.3983, 25.7177) (-53.4907, 25.6521) knots 0 0 0 1 2 2 2
  line L227 (-53.4907, 25.6521) -> (-53.4907, 24.05)
  line L228 (-53.4907, 24.05) -> (-54.2006, 24.05)
  line L229 (-54.2006, 24.05) -> (-54.2006, 25.1805)
  spline S139 degree 2 poles (-54.2006, 25.1805) (-54.2006, 25.3458) (-54.2152, 25.5767) (-54.2443, 25.6497) knots 0 0 0 1 2 2 2
  spline S140 degree 2 poles (-54.2443, 25.6497) (-54.2759, 25.7226) (-54.4024, 25.7882) (-54.5166, 25.7882) knots 0 0 0 1 2 2 2
  spline S141 degree 2 poles (-54.5166, 25.7882) (-54.6017, 25.7882) (-54.7694, 25.708) (-54.8472, 25.6521) knots 0 0 0 1 2 2 2
  line L230 (-54.8472, 25.6521) -> (-54.8472, 24.05)
  line L231 (-54.8472, 24.05) -> (-55.5523, 24.05)
  line L232 (-55.5523, 24.05) -> (-55.5523, 26.3134)
  line L233 (-55.5523, 26.3134) -> (-54.8472, 26.3134)
  line L234 (-54.8472, 26.3134) -> (-54.8472, 26.063)
  spline S142 degree 2 poles (-54.8472, 26.063) (-54.6746, 26.2088) (-54.3659, 26.3741) (-54.1738, 26.3741) knots 0 0 0 1 2 2 2
  spline S143 degree 2 poles (-54.1738, 26.3741) (-53.9672, 26.3741) (-53.6511, 26.1772) (-53.5685, 25.9803) knots 0 0 0 1 2 2 2
  spline S144 degree 2 poles (-53.5685, 25.9803) (-53.3667, 26.1699) (-53.0069, 26.3741) (-52.8221, 26.3741) knots 0 0 0 1 2 2 2
  spline S145 degree 2 poles (-52.8221, 26.3741) (-52.6641, 26.3741) (-52.4137, 26.2745) (-52.3286, 26.1724) knots 0 0 0 1 2 2 2
  spline S146 degree 2 poles (-52.3286, 26.1724) (-52.2338, 26.063) (-52.139, 25.7639) (-52.139, 25.5233) knots 0 0 0 1 2 2 2
  line L235 (-52.139, 25.5233) -> (-52.139, 24.05)
  line L236 (-52.139, 24.05) -> (-52.8489, 24.05)
  spline S147 degree 2 poles (-49.4453, 25.1805) (-49.4453, 24.6213) (-50.0555, 23.9795) (-50.6122, 23.9795) knots 0 0 0 1 2 2 2
  spline S148 degree 2 poles (-50.6122, 23.9795) (-51.1665, 23.9795) (-51.7816, 24.6213) (-51.7816, 25.1805) knots 0 0 0 1 2 2 2
  spline S149 degree 2 poles (-51.7816, 25.1805) (-51.7816, 25.7445) (-51.1665, 26.3839) (-50.6122, 26.3839) knots 0 0 0 1 2 2 2
  spline S150 degree 2 poles (-50.6122, 26.3839) (-50.0579, 26.3839) (-49.4453, 25.7421) (-49.4453, 25.1805) knots 0 0 0 1 2 2 2
  spline S151 degree 2 poles (-50.1673, 25.1756) (-50.1673, 25.3774) (-50.233, 25.6472) (-50.2913, 25.7275) knots 0 0 0 1 2 2 2
  spline S152 degree 2 poles (-50.2913, 25.7275) (-50.3545, 25.8126) (-50.5126, 25.8782) (-50.6122, 25.8782) knots 0 0 0 1 2 2 2
  spline S153 degree 2 poles (-50.6122, 25.8782) (-50.7095, 25.8782) (-50.8626, 25.8199) (-50.9259, 25.7372) knots 0 0 0 1 2 2 2
  spline S154 degree 2 poles (-50.9259, 25.7372) (-50.9866, 25.6594) (-51.0596, 25.3847) (-51.0596, 25.1756) knots 0 0 0 1 2 2 2
  spline S155 degree 2 poles (-51.0596, 25.1756) (-51.0596, 24.969) (-50.9915, 24.7137) (-50.9356, 24.6359) knots 0 0 0 1 2 2 2
  spline S156 degree 2 poles (-50.9356, 24.6359) (-50.8797, 24.5581) (-50.7095, 24.4852) (-50.6074, 24.4852) knots 0 0 0 1 2 2 2
  spline S157 degree 2 poles (-50.6074, 24.4852) (-50.5223, 24.4852) (-50.3472, 24.5581) (-50.2938, 24.631) knots 0 0 0 1 2 2 2
  spline S158 degree 2 poles (-50.2938, 24.631) (-50.233, 24.7161) (-50.1673, 24.9617) (-50.1673, 25.1756) knots 0 0 0 1 2 2 2
  spline S159 degree 2 poles (-48.2054, 24.0062) (-48.6357, 24.0062) (-49.0296, 24.3612) (-49.0296, 24.7647) knots 0 0 0 1 2 2 2
  line L237 (-49.0296, 24.7647) -> (-49.0296, 25.8223)
  line L238 (-49.0296, 25.8223) -> (-49.2994, 25.8223)
  line L239 (-49.2994, 25.8223) -> (-49.2994, 26.3134)
  line L240 (-49.2994, 26.3134) -> (-49.0296, 26.3134)
  line L241 (-49.0296, 26.3134) -> (-49.0296, 26.96)
  line L242 (-49.0296, 26.96) -> (-48.3246, 26.96)
  line L243 (-48.3246, 26.96) -> (-48.3246, 26.3134)
  line L244 (-48.3246, 26.3134) -> (-47.6438, 26.3134)
  line L245 (-47.6438, 26.3134) -> (-47.6438, 25.8223)
  line L246 (-47.6438, 25.8223) -> (-48.3246, 25.8223)
  line L247 (-48.3246, 25.8223) -> (-48.3246, 25.0176)
  spline S160 degree 2 poles (-48.3246, 25.0176) (-48.3246, 24.8985) (-48.3197, 24.721) (-48.2905, 24.6505) knots 0 0 0 1 2 2 2
  spline S161 degree 2 poles (-48.2905, 24.6505) (-48.2613, 24.58) (-48.1179, 24.4973) (-47.9818, 24.4973) knots 0 0 0 1 2 2 2
  spline S162 degree 2 poles (-47.9818, 24.4973) (-47.9234, 24.4973) (-47.7411, 24.5459) (-47.7046, 24.5654) knots 0 0 0 1 2 2 2
  line L248 (-47.7046, 24.5654) -> (-47.6438, 24.5654)
  line L249 (-47.6438, 24.5654) -> (-47.6438, 24.0694)
  spline S163 degree 2 poles (-47.6438, 24.0694) (-47.7581, 24.0403) (-48.0158, 24.0062) (-48.2054, 24.0062) knots 0 0 0 1 2 2 2
  spline S164 degree 2 poles (-46.1973, 23.9892) (-46.8391, 23.9892) (-47.5223, 24.6019) (-47.5223, 25.1683) knots 0 0 0 1 2 2 2
  spline S165 degree 2 poles (-47.5223, 25.1683) (-47.5223, 25.7226) (-46.8853, 26.3839) (-46.3116, 26.3839) knots 0 0 0 1 2 2 2
  spline S166 degree 2 poles (-46.3116, 26.3839) (-45.7938, 26.3839) (-45.2686, 25.8223) (-45.2686, 25.302) knots 0 0 0 1 2 2 2
  line L250 (-45.2686, 25.302) -> (-45.2686, 25.0468)
  line L251 (-45.2686, 25.0468) -> (-46.8173, 25.0468)
  spline S167 degree 2 poles (-46.8173, 25.0468) (-46.8075, 24.8887) (-46.6933, 24.6797) (-46.6009, 24.6165) knots 0 0 0 1 2 2 2
  spline S168 degree 2 poles (-46.6009, 24.6165) (-46.5109, 24.5532) (-46.2678, 24.4998) (-46.1244, 24.4998) knots 0 0 0 1 2 2 2
  spline S169 degree 2 poles (-46.1244, 24.4998) (-46.0028, 24.4998) (-45.7646, 24.5532) (-45.6649, 24.5994) knots 0 0 0 1 2 2 2
  spline S170 degree 2 poles (-45.6649, 24.5994) (-45.5774, 24.6359) (-45.4315, 24.7259) (-45.3853, 24.7599) knots 0 0 0 1 2 2 2
  line L252 (-45.3853, 24.7599) -> (-45.31, 24.7599)
  line L253 (-45.31, 24.7599) -> (-45.31, 24.1764)
  spline S171 degree 2 poles (-45.31, 24.1764) (-45.3975, 24.1424) (-45.5385, 24.084) (-45.6649, 24.0549) knots 0 0 0 1 2 2 2
  spline S172 degree 2 poles (-45.6649, 24.0549) (-45.7792, 24.0233) (-46.0223, 23.9892) (-46.1973, 23.9892) knots 0 0 0 1 2 2 2
  spline S173 degree 2 poles (-45.9639, 25.4722) (-45.9688, 25.6959) (-46.1657, 25.9317) (-46.3675, 25.9317) knots 0 0 0 1 2 2 2
  spline S174 degree 2 poles (-46.3675, 25.9317) (-46.5741, 25.9317) (-46.8075, 25.6837) (-46.8197, 25.4722) knots 0 0 0 1 2 2 2
  line L254 (-46.8197, 25.4722) -> (-45.9639, 25.4722)
  spline S175 degree 2 poles (-42.3635, 23.9917) (-43.0393, 23.9917) (-43.8318, 24.8085) (-43.8318, 25.5476) knots 0 0 0 1 2 2 2
  spline S176 degree 2 poles (-43.8318, 25.5476) (-43.8318, 26.2599) (-43.0369, 27.1083) (-42.361, 27.1083) knots 0 0 0 1 2 2 2
  spline S177 degree 2 poles (-42.361, 27.1083) (-42.1835, 27.1083) (-41.8967, 27.067) (-41.7654, 27.033) knots 0 0 0 1 2 2 2
  spline S178 degree 2 poles (-41.7654, 27.033) (-41.6633, 27.0014) (-41.4226, 26.8968) (-41.3472, 26.8579) knots 0 0 0 1 2 2 2
  line L255 (-41.3472, 26.8579) -> (-41.3472, 26.1432)
  line L256 (-41.3472, 26.1432) -> (-41.4226, 26.1432)
  spline S179 degree 2 poles (-41.4226, 26.1432) (-41.4785, 26.1918) (-41.6438, 26.328) (-41.7484, 26.3912) knots 0 0 0 1 2 2 2
  spline S180 degree 2 poles (-41.7484, 26.3912) (-41.8529, 26.4568) (-42.1033, 26.5468) (-42.2419, 26.5468) knots 0 0 0 1 2 2 2
  spline S181 degree 2 poles (-42.2419, 26.5468) (-42.4048, 26.5468) (-42.6746, 26.4447) (-42.7986, 26.3158) knots 0 0 0 1 2 2 2
  spline S182 degree 2 poles (-42.7986, 26.3158) (-42.9105, 26.2015) (-43.0539, 25.8101) (-43.0539, 25.5451) knots 0 0 0 1 2 2 2
  spline S183 degree 2 poles (-43.0539, 25.5451) (-43.0539, 25.2656) (-42.9056, 24.8839) (-42.784, 24.7672) knots 0 0 0 1 2 2 2
  spline S184 degree 2 poles (-42.784, 24.7672) (-42.6673, 24.6529) (-42.3805, 24.5532) (-42.237, 24.5532) knots 0 0 0 1 2 2 2
  spline S185 degree 2 poles (-42.237, 24.5532) (-42.0887, 24.5532) (-41.8189, 24.6529) (-41.7265, 24.7137) knots 0 0 0 1 2 2 2
  spline S186 degree 2 poles (-41.7265, 24.7137) (-41.6244, 24.7745) (-41.4712, 24.9033) (-41.4153, 24.9544) knots 0 0 0 1 2 2 2
  line L257 (-41.4153, 24.9544) -> (-41.3472, 24.9544)
  line L258 (-41.3472, 24.9544) -> (-41.3472, 24.2494)
  spline S187 degree 2 poles (-41.3472, 24.2494) (-41.4299, 24.2105) (-41.6463, 24.1132) (-41.763, 24.0792) knots 0 0 0 1 2 2 2
  spline S188 degree 2 poles (-41.763, 24.0792) (-41.904, 24.0354) (-42.1495, 23.9917) (-42.3635, 23.9917) knots 0 0 0 1 2 2 2
  spline S189 degree 2 poles (-38.7727, 25.1805) (-38.7727, 24.6213) (-39.3829, 23.9795) (-39.9396, 23.9795) knots 0 0 0 1 2 2 2
  spline S190 degree 2 poles (-39.9396, 23.9795) (-40.4939, 23.9795) (-41.109, 24.6213) (-41.109, 25.1805) knots 0 0 0 1 2 2 2
  spline S191 degree 2 poles (-41.109, 25.1805) (-41.109, 25.7445) (-40.4939, 26.3839) (-39.9396, 26.3839) knots 0 0 0 1 2 2 2
  spline S192 degree 2 poles (-39.9396, 26.3839) (-39.3853, 26.3839) (-38.7727, 25.7421) (-38.7727, 25.1805) knots 0 0 0 1 2 2 2
  spline S193 degree 2 poles (-39.4947, 25.1756) (-39.4947, 25.3774) (-39.5604, 25.6472) (-39.6187, 25.7275) knots 0 0 0 1 2 2 2
  spline S194 degree 2 poles (-39.6187, 25.7275) (-39.6819, 25.8126) (-39.84, 25.8782) (-39.9396, 25.8782) knots 0 0 0 1 2 2 2
  spline S195 degree 2 poles (-39.9396, 25.8782) (-40.0369, 25.8782) (-40.19, 25.8199) (-40.2532, 25.7372) knots 0 0 0 1 2 2 2
  spline S196 degree 2 poles (-40.2532, 25.7372) (-40.314, 25.6594) (-40.387, 25.3847) (-40.387, 25.1756) knots 0 0 0 1 2 2 2
  spline S197 degree 2 poles (-40.387, 25.1756) (-40.387, 24.969) (-40.3189, 24.7137) (-40.263, 24.6359) knots 0 0 0 1 2 2 2
  spline S198 degree 2 poles (-40.263, 24.6359) (-40.207, 24.5581) (-40.0369, 24.4852) (-39.9348, 24.4852) knots 0 0 0 1 2 2 2
  spline S199 degree 2 poles (-39.9348, 24.4852) (-39.8497, 24.4852) (-39.6746, 24.5581) (-39.6212, 24.631) knots 0 0 0 1 2 2 2
  spline S200 degree 2 poles (-39.6212, 24.631) (-39.5604, 24.7161) (-39.4947, 24.9617) (-39.4947, 25.1756) knots 0 0 0 1 2 2 2
  line L259 (-36.2808, 24.05) -> (-36.9907, 24.05)
  line L260 (-36.9907, 24.05) -> (-36.9907, 25.1707)
  spline S201 degree 2 poles (-36.9907, 25.1707) (-36.9907, 25.3093) (-37.0126, 25.5816) (-37.0417, 25.6448) knots 0 0 0 1 2 2 2
  spline S202 degree 2 poles (-37.0417, 25.6448) (-37.0782, 25.7226) (-37.2143, 25.7882) (-37.331, 25.7882) knots 0 0 0 1 2 2 2
  spline S203 degree 2 poles (-37.331, 25.7882) (-37.4161, 25.7882) (-37.5936, 25.7226) (-37.6933, 25.6521) knots 0 0 0 1 2 2 2
  line L261 (-37.6933, 25.6521) -> (-37.6933, 24.05)
  line L262 (-37.6933, 24.05) -> (-38.3983, 24.05)
  line L263 (-38.3983, 24.05) -> (-38.3983, 26.3134)
  line L264 (-38.3983, 26.3134) -> (-37.6933, 26.3134)
  line L265 (-37.6933, 26.3134) -> (-37.6933, 26.063)
  spline S204 degree 2 poles (-37.6933, 26.063) (-37.5207, 26.2088) (-37.1925, 26.3741) (-36.9931, 26.3741) knots 0 0 0 1 2 2 2
  spline S205 degree 2 poles (-36.9931, 26.3741) (-36.6479, 26.3741) (-36.2808, 25.9365) (-36.2808, 25.5233) knots 0 0 0 1 2 2 2
  line L266 (-36.2808, 25.5233) -> (-36.2808, 24.05)
  spline S206 degree 2 poles (-34.8926, 24.0062) (-35.3229, 24.0062) (-35.7168, 24.3612) (-35.7168, 24.7647) knots 0 0 0 1 2 2 2
  line L267 (-35.7168, 24.7647) -> (-35.7168, 25.8223)
  line L268 (-35.7168, 25.8223) -> (-35.9866, 25.8223)
  line L269 (-35.9866, 25.8223) -> (-35.9866, 26.3134)
  line L270 (-35.9866, 26.3134) -> (-35.7168, 26.3134)
  line L271 (-35.7168, 26.3134) -> (-35.7168, 26.96)
  line L272 (-35.7168, 26.96) -> (-35.0117, 26.96)
  line L273 (-35.0117, 26.96) -> (-35.0117, 26.3134)
  line L274 (-35.0117, 26.3134) -> (-34.331, 26.3134)
  line L275 (-34.331, 26.3134) -> (-34.331, 25.8223)
  line L276 (-34.331, 25.8223) -> (-35.0117, 25.8223)
  line L277 (-35.0117, 25.8223) -> (-35.0117, 25.0176)
  spline S207 degree 2 poles (-35.0117, 25.0176) (-35.0117, 24.8985) (-35.0069, 24.721) (-34.9777, 24.6505) knots 0 0 0 1 2 2 2
  spline S208 degree 2 poles (-34.9777, 24.6505) (-34.9485, 24.58) (-34.8051, 24.4973) (-34.669, 24.4973) knots 0 0 0 1 2 2 2
  spline S209 degree 2 poles (-34.669, 24.4973) (-34.6106, 24.4973) (-34.4283, 24.5459) (-34.3918, 24.5654) knots 0 0 0 1 2 2 2
  line L278 (-34.3918, 24.5654) -> (-34.331, 24.5654)
  line L279 (-34.331, 24.5654) -> (-34.331, 24.0694)
  spline S210 degree 2 poles (-34.331, 24.0694) (-34.4453, 24.0403) (-34.703, 24.0062) (-34.8926, 24.0062) knots 0 0 0 1 2 2 2
  line L280 (-32.5247, 25.6448) -> (-32.5831, 25.6448)
  spline S211 degree 2 poles (-32.5831, 25.6448) (-32.6244, 25.6594) (-32.7776, 25.674) (-32.8699, 25.674) knots 0 0 0 1 2 2 2
  spline S212 degree 2 poles (-32.8699, 25.674) (-32.9793, 25.674) (-33.2249, 25.6083) (-33.3391, 25.5646) knots 0 0 0 1 2 2 2
  line L281 (-33.3391, 25.5646) -> (-33.3391, 24.05)
  line L282 (-33.3391, 24.05) -> (-34.0442, 24.05)
  line L283 (-34.0442, 24.05) -> (-34.0442, 26.3134)
  line L284 (-34.0442, 26.3134) -> (-33.3391, 26.3134)
  line L285 (-33.3391, 26.3134) -> (-33.3391, 25.9876)
  spline S213 degree 2 poles (-33.3391, 25.9876) (-33.2905, 26.0314) (-33.1203, 26.1675) (-33.0498, 26.2088) knots 0 0 0 1 2 2 2
  spline S214 degree 2 poles (-33.0498, 26.2088) (-32.972, 26.255) (-32.7678, 26.3207) (-32.6779, 26.3207) knots 0 0 0 1 2 2 2
  spline S215 degree 2 poles (-32.6779, 26.3207) (-32.6438, 26.3207) (-32.5588, 26.3158) (-32.5247, 26.3134) knots 0 0 0 1 2 2 2
  line L286 (-32.5247, 26.3134) -> (-32.5247, 25.6448)
  spline S216 degree 2 poles (-30.0839, 25.1805) (-30.0839, 24.6213) (-30.6941, 23.9795) (-31.2508, 23.9795) knots 0 0 0 1 2 2 2